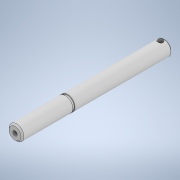
# Autodesk Inventor part: 10mmPins
Saved by Autodesk Inventor 2022 (Build 260153000, 153)
## iProperties
Created: 2022-05-04
Part Number: 10mmPins
Material: Generic
Document SubType Name: Modeling
Designer: Patrick
Density: 1 g/cm^3
Appearance: Default
Author: Patrick
Autodesk Inventor part; units mm, degrees
ref_plane "YZ Plane" through (0, 0, 0) normal (1, 0, 0) x (0, 1, 0)
ref_plane "XY Plane" through (0, 0, 0) normal (0, 0, 1) x (1, 0, 0)
sketch "Sketch1" plane through (0, 0, 0) normal (0, 1, 0) x (-1, 0, 0)
  line L0 (0, 0) -> (5, 0)
  line L1 (5, 0) -> (5, -100)
  line L2 (5, -100) -> (0, -100)
  line L3 (0, -100) -> (0, 0)
  line L4 (5, -33.5) -> (4.5, -33.5)
  line L5 (4.5, -33.5) -> (4.5, -35)
  line L6 (4.5, -35) -> (5, -35)
  line L7 (5, -35) -> (5, -33.5)
  line L8 (5, -90) -> (0, -90) construction
  line L9 (5, -99.003) -> (4.003, -100)
  line L10 (4, 0) -> (5, -1)
  dimension "d0" = 5
  dimension "d1" = 100
  dimension "d2" = 1.5
  dimension "d3" = 0.5
  dimension "d4" = 135
  dimension "d5" = 10
  dimension "d6" = 55
  dimension "d7" = 1.41
  dimension "d8" = 45
  dimension "d9" = 1.4142
  constraints: 22 end point, 7 point on line, 4 parallel, 3 perpendicular, 2 horizontal
  measures "d0" distance of L1.end L2.end
  measures "d1" distance of L0.end L1.end
  measures "d2" distance of L4.end L5.end
  measures "d3" distance of L5.end L6.end
  measures "d4" angle of L1 L9
  measures "d5" distance between parallel lines of L8 L2
  measures "d6" distance between parallel lines of L6 L8
  measures "d7" distance of L9.start L9.end
  measures "d8" angle of L0 L10
  measures "d9" distance of L10.start L10.end
revolve "Revolution1" add sketch "Sketch1" angle 360 about axis through (0, 0, -100) along (0, 0, 1) contours L0 L10 L1 L4 L5 L6 L9 L2 L3
ref_plane "Work Plane1" through (0, 5, -67.0015) normal (0, 1, 0) x (-1, 0, 0)
sketch "Sketch2" plane through (0, 5, -67.0015) normal (0, 1, 0) x (-1, 0, 0)
  circle A0 centre (0, -29.9985) radius 1.75
  line L0 (-4.003, -32.9985) -> (4.003, -32.9985) projected
  point P0 (0, 67.0015)
  dimension "d11" = 3.5
  dimension "d12" = 3
  constraints: 1 centre point
  measures "d11" diameter of A0
  measures "d12" distance from line of A0.centre L0
extrude "Extrusion1" cut sketch "Sketch2" against normal blind 10
sketch "Sketch3" plane through (0, 0, 0) normal (0, 0, 1) x (1, 0, 0)
  circle A0 centre (0, 0) radius 1.5
  dimension "d15" = 3
  constraints: 1 centre point, 1 coincident
  measures "d15" diameter of A0
extrude "Extrusion2" cut sketch "Sketch3" against normal blind 10
thread "Thread1" size "M3x0.5" class "6H" standard "ANSI Metric M Profile" length 10
body "Solid1"
